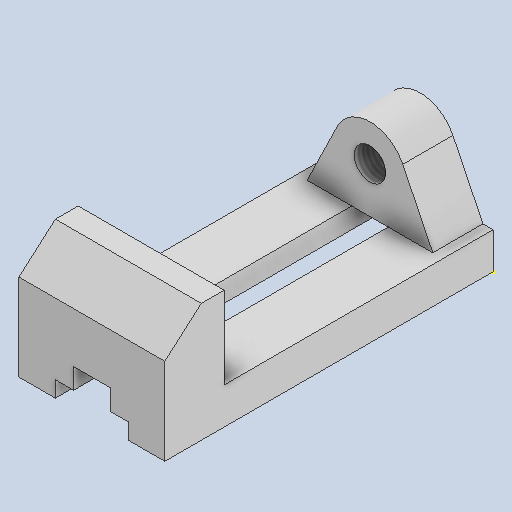
# Autodesk Inventor part: morsa_body
Saved by Autodesk Inventor 2022 (Build 260153000, 153)
## iProperties
Created: 2022-03-09
Part Number: morsa_body
Material: Genérico
Document SubType Name: Modeling
Designer: 19710060
Density: 1 g/cm^3
Appearance: Padrão
Author: 19710060
Autodesk Inventor part; units mm, degrees
ref_plane "YZ Plane" through (0, 0, 0) normal (1, 0, 0) x (0, 1, 0)
ref_plane "XZ Plane" through (0, 0, 0) normal (0, 1, 0) x (-1, 0, 0)
ref_plane "XY Plane" through (0, 0, 0) normal (0, 0, 1) x (1, 0, 0)
sketch "Esboço1" plane through (0, 0, 0) normal (1, 0, 0) x (0, 1, 0)
  line L0 (0, 0) -> (0, -144)
  line L1 (0, -144) -> (52, -144)
  line L2 (52, -144) -> (52, -122)
  line L3 (52, -122) -> (16, -122)
  line L4 (0, 0) -> (38, 0)
  line L5 (38, 0) -> (52, 0)
  line L6 (16, -122) -> (16, -26)
  line L7 (16, -26) -> (52, -26)
  line L8 (52, -26) -> (52, -16)
  line L9 (52, -16) -> (38, 0)
  dimension "d0" = 144
  dimension "d1" = 52
  dimension "d2" = 22
  dimension "d3" = 36
  dimension "d8" = 38
  dimension "d10" = 96
  dimension "d12" = 10
  constraints: 20 end point, 4 perpendicular, 3 vertical, 2 horizontal
  measures "d0" distance of L0.start L0.end
  measures "d1" distance of L0.end L1.end
  measures "d2" distance of L1.end L2.end
  measures "d3" distance of L2.end L3.end
  measures "d8" distance of L0.start L4.end
  measures "d10" distance of L3.end L6.end
  measures "d12" distance of L7.end L8.end
extrude "Extrusão1" add sketch "Esboço1" against normal blind 64
sketch "Esboço2" plane through (0, 0, -144) normal (0, 0, -1) x (-1, 0, 0)
  line L0 (0, 0) -> (16, 0)
  line L1 (0, 0) -> (64, 0) projected
  line L2 (16, 0) -> (16, 7)
  line L3 (16, 7) -> (24, 7)
  line L4 (24, 7) -> (24, 16)
  line L5 (24, 16) -> (40, 16)
  line L6 (0, 16) -> (64, 16) projected
  line L7 (40, 16) -> (40, 7)
  line L8 (40, 7) -> (48, 7)
  line L9 (48, 7) -> (48, 0)
  dimension "d15" = 16
  dimension "d16" = 7
  dimension "d20" = 16
  dimension "d21" = 9
  dimension "d22" = 8
  constraints: 16 end point, 4 perpendicular, 3 point on line, 2 vertical
  measures "d15" distance of L0.start L0.end
  measures "d16" distance of L0.end L2.end
  measures "d20" distance of L4.end L5.end
  measures "d21" distance of L5.end L7.end
  measures "d22" distance of L7.end L8.end
extrude "Extrusão2" cut sketch "Esboço2" against normal blind 144
sketch "Esboço3" plane through (0, 0, -144) normal (0, 0, -1) x (-1, 0, 0)
  point P0 (0, 0)
sketch "Esboço5" plane through (0, 0, -144) normal (0, 0, -1) x (-1, 0, 0)
  line L0 (48, 0) -> (64, 0) projected
  line L1 (0, 52) -> (64, 52) projected
  line L2 (64, 52) -> (64, 0) projected
  line L3 (40, 16) -> (64, 16) projected
  line L4 (24, 16) -> (40, 16) projected
  circle A0 centre (32, 36) radius 16
  line L5 (46.3807, 43.0139) -> (59.5563, 16)
  line L6 (17.6193, 43.0139) -> (4.4437, 16)
  line L7 (0, 0) -> (0, 52) projected
  line L8 (0, 0) -> (0, 16)
  line L9 (0, 16) -> (4.4437, 16)
  line L10 (0, 16) -> (24, 16) projected
  line L11 (59.5563, 16) -> (64, 16)
  line L12 (64, 16) -> (64, 0)
  point P0 (32, 52)
  constraints: 12 end point, 3 collinear, 2 point on circle, 2 point on line, 2 tangent, 1 centre point, 1 perpendicular
extrude "Extrusão3" cut sketch "Esboço5" against normal blind 22 contours L1 A0 L6 L9 L7 | L1 L2 L3 L5 A0
sketch "Esboço6" plane through (0, 0, -144) normal (0, 0, -1) x (-1, 0, 0)
  line L0 (24, 16) -> (40, 16) projected
  line L1 (32, 16) -> (32, 36)
  point P0 (0, 0)
  dimension "d49" = 20
  constraints: 2 end point, 1 midpoint, 1 vertical
  measures "d49" distance of L1.start L1.end
hole "Furo1" at (-32, 36, -144) direction (0, 0, 1) diameter 13.835 depth 22 tip angle 118 thread size "M16x2" class "6H" standard "ISO Metric profile"
sketch "Esboço7" plane through (-64, 0, -144) normal (0, -1, 0) x (1, 0, 0)
  line L0 (0, 144) -> (0, 128) projected
  line L1 (10, 108) -> (10, 36)
  line L2 (54, 108) -> (54, 36)
  point P0 (64, 144)
  dimension "d59" = 72
  dimension "d61" = 72
  constraints: 4 end point
  measures "d59" distance of L1.start L1.end
  measures "d61" distance of L2.start L2.end
hole "Furo2" at (-10, 0, -36) at (-10, 0, -108) at (-54, 0, -108) at (-54, 0, -36) direction (0, 1, 0) diameter 4.917 depth 12 tip angle 118 thread size "M6x1" class "6H" standard "ISO Metric profile"
